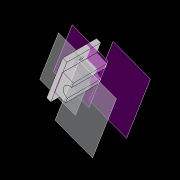
# Autodesk Inventor part: Soporte Superior Tubos
Saved by Autodesk Inventor 2021 (Build 250183000, 183)
## iProperties
Created: 2021-05-02
Part Number: Soporte Superior Tubos
Material: Generic
Document SubType Name: Modeling
Designer: maaro
Density: 1 g/cm^3
Appearance: Default
Author: maaro
Autodesk Inventor part; units mm, degrees
ref_plane "YZ Plane" through (0, 0, 0) normal (1, 0, 0) x (0, 1, 0)
ref_plane "XZ Plane" through (0, 0, 0) normal (0, 1, 0) x (-1, 0, 0)
ref_plane "XY Plane" through (0, 0, 0) normal (0, 0, 1) x (1, 0, 0)
ref_plane "Work Plane1" through (69.0193, -25.7667, -4444.0205) normal (0, 0, 1) x (0.3535607, 0.9354116, 0)
sketch "Sketch1" plane through (69.0193, -25.7667, -4444.0205) normal (0, 0, 1) x (0.3535607, 0.9354116, 0)
  circle A0 centre (-0.3, 73.6715) radius 26.9875 projected
  arc A1 (26.6875, 73.6715) -> (-27.2875, 73.6715) centre (-0.3, 73.6715) ccw
  line L0 (-0.3, 73.6715) -> (49.7, 73.6715) construction
  line L1 (-0.3, 73.6715) -> (-50.3, 73.6715) construction
  line L2 (-27.2875, 73.6715) -> (-50.3, 73.6715)
  line L3 (-50.3, 73.6715) -> (-50.3, 123.6715)
  line L4 (-50.3, 123.6715) -> (49.7, 123.6715)
  line L5 (49.7, 123.6715) -> (49.7, 73.6715)
  line L6 (49.7, 73.6715) -> (26.6875, 73.6715)
  point P0 (-0.3, 73.6715)
  dimension "d1" = 180
  dimension "d2" = 50
  dimension "d3" = 100
  dimension "d4" = 50
  constraints: 14 end point, 4 point on circle, 2 coincident, 2 collinear, 2 perpendicular, 1 centre point, 1 concentric, 1 horizontal, 1 vertical
  measures "d1" angle of L1 L0
  measures "d2" distance of L4.end L0.end
  measures "d3" distance between parallel lines of L5 L3
  measures "d4" distance from line of point (-0.3, 73.672) L3
ref_plane "Work Plane2" through (69.0193, -25.7667, -4594.0205) normal (0, 0, -1) x (-0.3535607, -0.9354116, 0)
extrude "Extrusion1" add sketch "Sketch1" against normal up to surface (150 mm away) contours A0 L2 L3 L4 L5 L6
ref_plane "Work Plane3" through (-64.4486, -29.0925, -4594.0205) normal (-0.9354116, 0.3535607, 0) x (0, 0, 1)
sketch "Sketch2" plane through (-64.4486, -29.0925, -4594.0205) normal (-0.9354116, 0.3535607, 0) x (0, 0, 1)
  line L0 (150, -49.7) -> (0, -49.7) projected
  line L1 (150, 150.3) -> (0, 150.3) projected
  line L2 (0, -49.7) -> (0, 150.3)
  line L3 (150, -49.7) -> (150, 150.3)
  circle A0 centre (75, 120.3) radius 7.5 projected
  circle A1 centre (75, -19.7) radius 7.5 projected
  point P0 (4594.0205, 50)
  constraints: 4 end point, 1 parallel, 1 vertical
extrude "Extrusion2" add sketch "Sketch2" along normal blind 20 separate body
ref_plane "Work Plane5" through (-82.0206, -75.5825, -4489.0205) normal (0, 0, 1) x (0.9354116, -0.3535607, 0)
ref_plane "Work Plane6" through (-82.0206, -75.5825, -4549.0205) normal (0, 0, -1) x (-0.9354116, 0.3535607, 0)
sketch "Sketch3" plane through (-82.0206, -75.5825, -4489.0205) normal (0, 0, 1) x (0.9354116, -0.3535607, 0)
  line L0 (-20, 200) -> (-20, 0) projected
  line L1 (50, 49.7) -> (50, 72.7125) projected
  line L2 (50, 126.6875) -> (50, 149.7) projected
  line L3 (-20, 0) -> (-20, 200) projected
  line L4 (-20, 73.0125) -> (-31, 73.0125)
  line L5 (-31, 73.0125) -> (-31, 126.9875)
  line L6 (-31, 126.9875) -> (-20, 126.9875)
  line L7 (-20, 78.0125) -> (-26, 78.0125)
  line L8 (-26, 78.0125) -> (-26, 121.9875)
  line L9 (-26, 121.9875) -> (-20, 121.9875)
  line L10 (-20, 73.0125) -> (-20, 78.0125)
  line L11 (-20, 121.9875) -> (-20, 126.9875)
  line L12 (-31, 100) -> (-26, 100) construction
  line L13 (0, 0) -> (-20, 0) projected
  point P0 (50, 99.7)
  point P1 (-20, 73.0125)
  point P2 (-20, 78.0125)
  point P3 (-20, 121.9875)
  point P4 (-20, 126.9875)
  dimension "d14" = 5
  dimension "d15" = 100
  dimension "d16" = 11
  dimension "d17" = 26.9875
  constraints: 18 end point, 4 perpendicular, 2 midpoint, 2 point on line, 1 collinear, 1 vertical, 2 other
  measures "d14" distance between parallel lines of L4 L7
  measures "d15" distance between parallel lines of L12 L13
  measures "d16" distance of L5.end L6.end
  measures "d17" distance between parallel lines of L12 L6
extrude "Extrusion3" add sketch "Sketch3" against normal up to surface (60 mm away) separate body contours L0 L9 L8 L7 L4 L5 L6
sketch "Sketch4" plane through (-85.204, 3.6746, -4549.0205) normal (-0.9354116, 0.3535607, 0) x (0, 0, 1)
  line L0 (60, 53.975) -> (60, 0) projected
  line L1 (60, 53.975) -> (0, 53.975) projected
  circle A0 centre (30, 26.6875) radius 5
  point P0 (4549.0205, 26.6875)
  dimension "d20" = 30
  dimension "d21" = 27.2875
  dimension "d22" = 10
  constraints: 1 centre point, 1 coincident
  measures "d20" distance from line of point (30, 26.687) L0
  measures "d21" distance from line of point (30, 26.687) L1
  measures "d22" diameter of A0
extrude "Extrusion4" cut sketch "Sketch4" against normal up to next bodies 3
sketch "Sketch5" plane through (-83.1568, -22.0213, -4594.0205) normal (-0.9354116, 0.3535607, 0) x (0, 0, 1)
  circle A0 centre (75, 50) radius 5 projected
  point P0 (4594.0205, 50)
  point P1 (75, 50)
  constraints: 1 coincident
hole "Hole1" at (-65.4788, 24.7492, -4519.0205) direction (0.9354116, -0.3535607, 0) diameter 10 depth 10 tip angle 118 bodies 2
body "Solid1"
body "Solid2"
body "Solid3"
